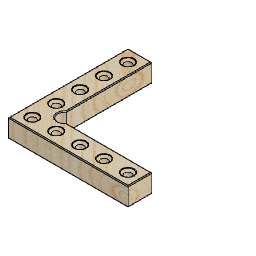
model (Autodesk Fusion 360 design; units mm, degrees)
Autodesk Fusion 360 part; units mm, degrees
sketch "Sketch1" plane through (0, 0, 0) normal (0, 0, 1) x (1, 0, 0) in component "square"
  line L0 (0, 160) -> (0, 0)
  line L1 (0, 0) -> (160, 0)
  line L2 (160, 0) -> (160, 32)
  line L3 (160, 32) -> (32, 32)
  line L4 (32, 32) -> (32, 160)
  line L5 (32, 160) -> (0, 160)
  line L6 (0, 0) -> (32, 32) construction
  line L7 (32, 160) -> (160, 32) construction
  line L8 (32, 32) -> (96, 96) construction
  circle A0 centre (16, 16) radius 4.7625
  line L9 (16, 16) -> (0, 16) construction
  line L10 (16, 16) -> (32, 16) construction
  circle A1 centre (16, 48) radius 4.7625
  circle A2 centre (16, 80) radius 4.7625
  circle A3 centre (16, 112) radius 4.7625
  circle A4 centre (16, 144) radius 4.7625
  line L11 (16, 16) -> (16, 0) construction
  circle A5 centre (48, 16) radius 4.7625
  circle A6 centre (80, 16) radius 4.7625
  circle A7 centre (112, 16) radius 4.7625
  circle A8 centre (144, 16) radius 4.7625
  line L12 (30.8775, 44.3479) -> (37.6127, 37.6127) construction
  line L13 (37.6127, 37.6127) -> (44.3479, 30.8775) construction
  circle A9 centre (37.6127, 37.6127) radius 9.525
  dimension "d6" = 32
  dimension "d7" = 160
  dimension "d8" = 9.525
  dimension "d12" = 0
  dimension "d13" = 128
  dimension "d16" = 128
  dimension "d17" = 0
  dimension "d22" = 32
  dimension "d33" = 19.05
  dimension "d34" = 7.9375
  constraint coincident L0.end L1.start
  constraint vertical L0
  constraint horizontal L5
  constraint vertical L4
  constraint vertical L2
  constraint horizontal L1
  constraint horizontal L3
  constraint perpendicular L6 L7
  constraint coincident L7 L8.end
  constraint collinear L6 L8
  constraint midpoint L7 L8.end
  constraint coincident A0.centre L9.start
  constraint coincident L0 L9.end
  constraint perpendicular L0 L9
  constraint coincident L4 L10.end
  constraint perpendicular L4 L10
  constraint equal L9 L10
  constraint coincident L1 L11.end
  constraint perpendicular L1 L11
  constraint equal L10 L11
  constraint coincident L8 L12.end
  constraint perpendicular L8 L12
  constraint collinear L12 L13
  constraint equal L12 L13
  constraint coincident L12.end L13.start
  constraint coincident L12.start A9
  measures "d6" distance of L0.start L4.end
  measures "d7" distance of L0.start L0.end
  measures "d8" diameter of A0
  measures "d22" distance of A3.centre A4.centre
  measures "d33" diameter of A9
  measures "d34" distance of L3.end L12.end
extrude "Extrude1" add sketch "Sketch1" along normal blind 25 contours L0 L1 L2 L3 L4 L5 A9 in component "square"
chamfer "Chamfer1" distance 3 angle 45 9 faces at (20.7388, 15.5258, 8.3333) (52.7388, 15.5258, 8.3333) (84.7388, 15.5258, 8.3333) (116.7388, 15.5258, 8.3333) (143.8813, 20.761, 16.6667) (20.7388, 47.5258, 8.3333) (11.8175, 77.7223, 16.6667) (20.6681, 111.0563, 16.6667) (11.3848, 142.8248, 16.6667) in component "square"
fillet "Fillet1" radius 1 2 faces at (21.3775, 32.7706, 25) (21.3775, 32.7706, 0) in component "square"
component "square" placed x (1, 0, 0) y (0, 1, 0) z (0, 0, 1) at (0, 0, 0)
equation "squareWidth = 32 mm"
equation "squareHeight = 160 mm"
equation "squareThickness = 25 mm"
equation "clampDiameter = 8 mm"
equation "squareHoleSize = 3 / 8 * 1\""
equation "d6 = squareWidth"
equation "d7 = squareHeight"
equation "d8 = squareHoleSize"
equation "squareHoleCount = 5"
equation "d11 = squareHoleCount"
equation "d13 = squareHeight - squareWidth"
equation "d14 = squareHoleCount"
equation "d16 = squareHeight - squareWidth"
equation "d23 = squareThickness"
equation "chamferSize = 3 mm"
equation "d26 = chamferSize"
equation "reliefDiameter = 3 / 4 * 1 in"
equation "reliefDepth = reliefDiameter / 2 / 6"
equation "d33 = reliefDiameter"
equation "d34 = reliefDiameter / 2 - reliefDepth"
